Autodesk Fusion 360 part; units mm, degrees
(part 2 of 3)
  measures "d264" distance of L157.end L157.start
  measures "d265" distance of L181.start L179.start
  measures "d266" distance of L180.end L182.end
  measures "d267" distance of L180.start L179.end
  measures "d268" distance of L154.end L154.start
  measures "d269" distance of L174.end L171.start
  measures "d270" distance of L153.start L154.end
  measures "d271" distance of L162.end L156.end
  measures "d272" distance of L156.start L156.end
  measures "d273" distance of L156 L187
  measures "d274" distance of L159.start L161.end
  measures "d275" distance of L158 L163
  measures "d276" distance of L158.end L153.end
  measures "d277" distance of L162.end L168.end
  measures "d278" distance of L157.end L165.end
  measures "d279" distance of L167.start L167.end
  measures "d280" distance of L190.end L189.end
  measures "d281" distance of L190.end L191.end
  measures "d282" distance of L194.start L195.end
  measures "d283" distance of L193.start L194.start
  measures "d284" distance of L192 L196
  measures "d285" distance of L187 L194
  measures "d286" distance of P0 L196
  measures "d287" distance of L200.start L197.end
  measures "d288" distance of L200.end L200.start
  measures "d289" distance of L198.start L198.end
  measures "d290" distance of L198.end L199.start
  measures "d291" distance of L198 L203
  measures "d292" distance of L205.end L207.end
  measures "d293" distance of L206.start L207.end
  measures "d294" distance of L202 L206
  measures "d295" distance of L212.end L214.end
  measures "d296" distance of L216.start L214.end
  measures "d297" distance of L217.start L215.end
  measures "d298" distance of L217.end L217.start
  measures "d300" distance of L210.end L209.start
  measures "d301" distance of L209.end L209.start
  measures "d303" distance of L200 L212
  measures "d305" distance of L156 L197
  measures "d306" distance of L221.end L221.start
  measures "d307" distance of L221.end L223.start
  measures "d312" distance of L242.end L237.end
  measures "d313" distance of L236.end L237.end
  measures "d314" distance of L236.end L236.start
  measures "d315" distance of L238.start L255.start
  measures "d316" distance of L241.end L244.start
  measures "d317" distance of L243.end L250.end
  measures "d318" distance of L239.end L239.start
  measures "d319" distance of L230.end L225.start
  measures "d320" distance of L229.start L232.start
  measures "d321" distance of L225.end L225.start
  measures "d322" distance of L249.start L231.end
  measures "d323" distance of L231.end L231.start
  measures "d324" distance of L231 L245
  measures "d325" distance of L234.end L236.start
  measures "d326" distance of L248 L256
  measures "d327" distance of L226.end L234.start
  measures "d328" distance of L249.start L230.start
  measures "d329" distance of L238.start L238.end
  measures "d330" distance of L251.end L245.start
  measures "d375" distance of L272.start L267.end
  measures "d376" distance of L264.end L267.end
  measures "d377" distance of L264.end L264.start
  measures "d378" distance of L261.start L266.start
  measures "d379" distance of L274.start L274.end
  measures "d380" distance of L276.start L276.end
  measures "d381" distance of L283.end L277.end
  measures "d382" distance of L269.end L269.start
  measures "d383" distance of L284.start L284.end
  measures "d384" distance of L270.end L269.end
  measures "d385" distance of L262.end L262.start
  measures "d386" distance of L275.end L262.start
  measures "d387" distance of L289 L290
  measures "d388" distance of L264.start L265.start
  measures "d389" distance of L265 L268
  measures "d390" distance of L268.end L268.start
  measures "d391" distance of L262.end L271.end
  measures "d392" distance of L261.start L261.end
  measures "d393" distance of L263.end L289.start
  measures "d395" distance of origin L220
  measures "d399" angle of L30 L221
  measures "d401" distance of L221 L297
  measures "d402" distance of L30 P2
  measures "d403" distance of L29 P2
  measures "d404" distance of L297 P2
  measures "d405" distance of L223 L298
  measures "d407" angle of L223 L233
  measures "d408" distance of L231 P5
  measures "d409" distance of L240 P5
  measures "d410" distance of L298 P5
  measures "d411" distance of L231 P6
  measures "d412" distance of L260 P6
  measures "d413" distance of L289 L304
  measures "d414" distance of P6 L304
  measures "d415" distance of L127 L305
  measures "d416" distance of L132 L306
  measures "d418" angle of L248 L289
  measures "d419" distance of L289 L307
  measures "d420" distance of L293 L308
  measures "d421" distance of L306 L307.end
  measures "d423" distance of L8 L309
  measures "d424" distance of L63 L310
  measures "d494" angle of L87 L314
  measures "d496" distance of L213 L314
  measures "d497" distance of L77 P7
  measures "d498" distance of L218 L315
  measures "d499" distance of L195 L317
  measures "d512" distance of L224 L319
  measures "d543" diameter of A3
  measures "d544" diameter of A4
  measures "d545" diameter of A5
  measures "d546" diameter of A6
  measures "d547" diameter of A7
  measures "d548" diameter of A8
  measures "d550" diameter of A9
  measures "d551" diameter of A10
  measures "d553" diameter of A11
  measures "d554" diameter of A12
  measures "d555" diameter of A13
  measures "d556" diameter of A14
  measures "d557" distance of L314 A11.centre
  measures "d558" distance of L315 A13.centre
  measures "d587" diameter of A15
  measures "d588" diameter of A16
  measures "d589" diameter of A17
  measures "d590" diameter of A18
  measures "d591" diameter of A19
  measures "d592" diameter of A20
  measures "d593" diameter of A21
  measures "d594" diameter of A22
  measures "d595" diameter of A23
  measures "d596" diameter of A24
  measures "d597" diameter of A25
  measures "d598" diameter of A26
  measures "d599" diameter of A27
  measures "d600" diameter of A28
  measures "d601" diameter of A29
  measures "d602" diameter of A30
  measures "d603" diameter of A31
  measures "d604" diameter of A32
  measures "d605" diameter of A33
  measures "d606" diameter of A34
  measures "d607" diameter of A35
  measures "d608" diameter of A36
  measures "d609" diameter of A37
  measures "d610" diameter of A38
  measures "d611" angle of L309 L317
  measures "d617" angle of L190 L334
  measures "d618" angle of L193 L335
  measures "d620" vertical distance of A5.centre A7.centre
  measures "d621" distance of A5.centre L322
  measures "d645" diameter of A39
  measures "d649" diameter of A40
  measures "d651" diameter of A41
  measures "d653" diameter of A42
  measures "d655" diameter of A43
  measures "d657" diameter of A44
  measures "d661" diameter of A45
  measures "d662" diameter of A46
  measures "d663" diameter of A47
  measures "d664" diameter of A48
  measures "d665" diameter of A49
  measures "d666" diameter of A50
  measures "d667" diameter of A51
  measures "d668" diameter of A52
  measures "d669" diameter of A53
  measures "d670" diameter of A54
  measures "d671" diameter of A55
  measures "d672" diameter of A56
  measures "d705" diameter of A62
  measures "d706" diameter of A61
  measures "d707" diameter of A58
  measures "d708" diameter of A57
  measures "d709" diameter of A60
  measures "d710" diameter of A59
extrude "Platte Rechts" add sketch "Skizze1" along normal blind 2.7 contours L309 L310 L311 A0 L314 A1 A2 L318 | A15 | A16 | A17 | A18 | A19 | A20 | A21 | A22 | A23 | A24 | A25 | A26 | A27 | A28 | A29 | A30 | A31 | A32 | A33 | A34 | A35 | A36 | A37 | A38 | A45 | A46 | A47 | A48 | A49 | A50 | A51 | A52 | A53 | A54 | A55 | A56 makes body 1
extrude "Platte Mitte" add sketch "Skizze1" along normal blind 2.7 separate body contours L313 L314 L315 L316 L317 | A3 | A4 | A5 | A6 | A7 | A8 | A9 | A10 | A11 | A12 | A13 | A14 | A39 | A40 | A41 | A42 | A43 | A44 | A57 | A58 | A59 | A60 | A61 | A62 makes body 2
sketch "Skizze5" plane through (0, 0, 0) normal (1, 0, 0) x (0, 1, 0)
  line L0 (0, 12.7887) -> (160, 19.7745)
  line L1 (0, 1.75) -> (0, 22.5)
  line L2 (1.75, 0) -> (22.5, 0)
  point P0 (14, 13.4)
  dimension "d440" = 2.5
  dimension "d441" = 160
  dimension "d450" = 14
  dimension "d451" = 13.4
  constraint coincident L0.start L1
  constraint coincident L0 P0
  measures "d440" angle of L0 L2
  measures "d441" distance of L0.end L1
  measures "d450" distance of L1 P0
  measures "d451" distance of L2 P0
ref_plane "Arbeitsebene1" through (0, 80, 16.2816) normal (0, 0.043619, -0.999048) x (0, 0.999048, 0.043619)
sketch "Skizze4" plane through (0, 0, 2.7) normal (0, 0, 1) x (-1, 0, 0)
  line L0 (97.7927, -100.387) -> (100.2238, -86.5997)
  line L1 (100.2238, -86.5997) -> (114.0111, -89.0308)
  line L2 (114.0111, -89.0308) -> (111.58, -102.8181)
  line L3 (111.58, -102.8181) -> (97.7927, -100.387)
  line L4 (133.2058, -89.8768) -> (130.7747, -103.6641)
  line L5 (130.7747, -103.6641) -> (116.9874, -101.233)
  line L6 (116.9874, -101.233) -> (119.4185, -87.4457)
  line L7 (119.4185, -87.4457) -> (133.2058, -89.8768)
  line L8 (96.9158, -105.3603) -> (110.7031, -107.7914)
  line L9 (110.7031, -107.7914) -> (108.272, -121.5787)
  line L10 (108.272, -121.5787) -> (94.4847, -119.1476)
  line L11 (94.4847, -119.1476) -> (96.9158, -105.3603)
  line L12 (110.3714, -138.7542) -> (112.8025, -124.9669)
  line L13 (112.8025, -124.9669) -> (126.5898, -127.3979)
  line L14 (126.5898, -127.3979) -> (124.1587, -141.1852)
  line L15 (124.1587, -141.1852) -> (110.3714, -138.7542)
  line L16 (107.3951, -126.552) -> (104.964, -140.3393)
  line L17 (104.964, -140.3393) -> (91.1767, -137.9082)
  line L18 (91.1767, -137.9082) -> (93.6078, -124.1209)
  line L19 (93.6078, -124.1209) -> (107.3951, -126.552)
  line L20 (156.9327, -65.0193) -> (143.1454, -62.5882)
  line L21 (143.1454, -62.5882) -> (145.5765, -48.8009)
  line L22 (145.5765, -48.8009) -> (159.3638, -51.232)
  line L23 (159.3638, -51.232) -> (156.9327, -65.0193)
  line L24 (39.3317, -102.8224) -> (41.7627, -89.0351)
  line L25 (41.7627, -89.0351) -> (55.55, -91.4661)
  line L26 (55.55, -91.4661) -> (53.119, -105.2534)
  line L27 (53.119, -105.2534) -> (39.3317, -102.8224)
  line L28 (78.5893, -99.5903) -> (92.3766, -102.0214)
  line L29 (92.3766, -102.0214) -> (89.9455, -115.8087)
  line L30 (89.9455, -115.8087) -> (76.1582, -113.3776)
  line L31 (76.1582, -113.3776) -> (78.5893, -99.5903)
  line L32 (56.868, -113.0733) -> (70.6553, -115.5043)
  line L33 (70.6553, -115.5043) -> (68.2243, -129.2916)
  line L34 (68.2243, -129.2916) -> (54.437, -126.8606)
  line L35 (54.437, -126.8606) -> (56.868, -113.0733)
  line L36 (52.242, -110.2267) -> (49.811, -124.014)
  line L37 (49.811, -124.014) -> (36.0237, -121.583)
  line L38 (36.0237, -121.583) -> (38.4547, -107.7956)
  line L39 (38.4547, -107.7956) -> (52.242, -110.2267)
  line L40 (75.2813, -118.3509) -> (89.0686, -120.7819)
  line L41 (89.0686, -120.7819) -> (86.6376, -134.5693)
  line L42 (86.6376, -134.5693) -> (72.8502, -132.1382)
  line L43 (72.8502, -132.1382) -> (75.2813, -118.3509)
  line L44 (57.7449, -108.1) -> (60.176, -94.3127)
  line L45 (60.176, -94.3127) -> (73.9633, -96.7437)
  line L46 (73.9633, -96.7437) -> (71.5323, -110.5311)
  line L47 (71.5323, -110.5311) -> (57.7449, -108.1)
  line L48 (81.8973, -80.8297) -> (95.6846, -83.2608)
  line L49 (95.6846, -83.2608) -> (93.2535, -97.0481)
  line L50 (93.2535, -97.0481) -> (79.4662, -94.617)
  line L51 (79.4662, -94.617) -> (81.8973, -80.8297)
  line L52 (63.484, -75.5521) -> (77.2713, -77.9832)
  line L53 (77.2713, -77.9832) -> (74.8403, -91.7705)
  line L54 (74.8403, -91.7705) -> (61.0529, -89.3394)
  line L55 (61.0529, -89.3394) -> (63.484, -75.5521)
  line L56 (66.792, -56.7915) -> (80.5793, -59.2226)
  line L57 (80.5793, -59.2226) -> (78.1483, -73.0099)
  line L58 (78.1483, -73.0099) -> (64.3609, -70.5788)
  line L59 (64.3609, -70.5788) -> (66.792, -56.7915)
  line L60 (85.2053, -62.0691) -> (98.9926, -64.5002)
  line L61 (98.9926, -64.5002) -> (96.5615, -78.2875)
  line L62 (96.5615, -78.2875) -> (82.7742, -75.8564)
  line L63 (82.7742, -75.8564) -> (85.2053, -62.0691)
  line L64 (56.4175, -85.2219) -> (50.228, -84.1305)
  line L65 (50.228, -84.1305) -> (50.0847, -84.943)
  line L66 (50.0847, -84.943) -> (47.3421, -84.4594)
  line L67 (47.3421, -84.4594) -> (47.4853, -83.6469)
  line L68 (47.4853, -83.6469) -> (44.3044, -83.086)
  line L69 (44.3044, -83.086) -> (45.4765, -76.4386)
  line L70 (45.4765, -76.4386) -> (48.6574, -76.9995)
  line L71 (48.6574, -76.9995) -> (48.9223, -75.4976)
  line L72 (48.9223, -75.4976) -> (44.2937, -74.6815)
  line L73 (44.2937, -74.6815) -> (46.7247, -60.8942)
  line L74 (46.7247, -60.8942) -> (51.3533, -61.7103)
  line L75 (51.3533, -61.7103) -> (51.6181, -60.2085)
  line L76 (51.6181, -60.2085) -> (48.4372, -59.6476)
  line L77 (48.4372, -59.6476) -> (49.6093, -53.0002)
  line L78 (49.6093, -53.0002) -> (52.7903, -53.561)
  line L79 (52.7903, -53.561) -> (52.9335, -52.7486)
  line L80 (52.9335, -52.7486) -> (55.6762, -53.2322)
  line L81 (55.6762, -53.2322) -> (55.533, -54.0446)
  line L82 (55.533, -54.0446) -> (61.7225, -55.136)
  line L83 (61.7225, -55.136) -> (61.4229, -56.8348)
  line L84 (61.4229, -56.8348) -> (62.6047, -57.0432)
  line L85 (62.6047, -57.0432) -> (62.0317, -60.2931)
  line L86 (62.0317, -60.2931) -> (60.8499, -60.0847)
  line L87 (60.8499, -60.0847) -> (60.5503, -61.7835)
  line L88 (60.5503, -61.7835) -> (56.1483, -61.0073)
  line L89 (56.1483, -61.0073) -> (55.8834, -62.5091)
  line L90 (55.8834, -62.5091) -> (60.512, -63.3252)
  line L91 (60.512, -63.3252) -> (58.081, -77.1126)
  line L92 (58.081, -77.1126) -> (53.4524, -76.2964)
  line L93 (53.4524, -76.2964) -> (53.1876, -77.7982)
  line L94 (53.1876, -77.7982) -> (57.5896, -78.5744)
  line L95 (57.5896, -78.5744) -> (57.2901, -80.2732)
  line L96 (57.2901, -80.2732) -> (58.4719, -80.4816)
  line L97 (58.4719, -80.4816) -> (57.8988, -83.7315)
  line L98 (57.8988, -83.7315) -> (56.7171, -83.5231)
  line L99 (56.7171, -83.5231) -> (56.4175, -85.2219)
  line L100 (109.906, -37.6121) -> (123.0617, -42.4003)
  line L101 (123.0617, -42.4003) -> (118.2734, -55.556)
  line L102 (118.2734, -55.556) -> (105.1177, -50.7677)
  line L103 (105.1177, -50.7677) -> (109.906, -37.6121)
  line L104 (79.2965, -35.8234) -> (81.6465, -31.753)
  line L105 (81.6465, -31.753) -> (93.7709, -38.753)
  line L106 (93.7709, -38.753) -> (91.4209, -42.8234)
  line L107 (91.4209, -42.8234) -> (92.7416, -43.5859)
  line L108 (92.7416, -43.5859) -> (94.3566, -40.7886)
  line L109 (94.3566, -40.7886) -> (100.2022, -44.1636)
  line L110 (100.2022, -44.1636) -> (98.5872, -46.9609)
  line L111 (98.5872, -46.9609) -> (99.3017, -47.3734)
  line L112 (99.3017, -47.3734) -> (97.9092, -49.7852)
  line L113 (97.9092, -49.7852) -> (97.1947, -49.3727)
  line L114 (97.1947, -49.3727) -> (94.0522, -54.8157)
  line L115 (94.0522, -54.8157) -> (92.5583, -53.9532)
  line L116 (92.5583, -53.9532) -> (91.9583, -54.9924)
  line L117 (91.9583, -54.9924) -> (89.1005, -53.3424)
  line L118 (89.1005, -53.3424) -> (89.7005, -52.3032)
  line L119 (89.7005, -52.3032) -> (88.2066, -51.4407)
  line L120 (88.2066, -51.4407) -> (90.4416, -47.5696)
  line L121 (90.4416, -47.5696) -> (89.1209, -46.8071)
  line L122 (89.1209, -46.8071) -> (86.7709, -50.8774)
  line L123 (86.7709, -50.8774) -> (74.6465, -43.8774)
  line L124 (74.6465, -43.8774) -> (76.9965, -39.8071)
  line L125 (76.9965, -39.8071) -> (75.6758, -39.0446)
  line L126 (75.6758, -39.0446) -> (73.4408, -42.9157)
  line L127 (73.4408, -42.9157) -> (71.9469, -42.0532)
  line L128 (71.9469, -42.0532) -> (71.3469, -43.0924)
  line L129 (71.3469, -43.0924) -> (68.4891, -41.4424)
  line L130 (68.4891, -41.4424) -> (69.0891, -40.4032)
  line L131 (69.0891, -40.4032) -> (67.5952, -39.5407)
  line L132 (67.5952, -39.5407) -> (70.7377, -34.0977)
  line L133 (70.7377, -34.0977) -> (70.0232, -33.6852)
  line L134 (70.0232, -33.6852) -> (71.4157, -31.2734)
  line L135 (71.4157, -31.2734) -> (72.1302, -31.6859)
  line L136 (72.1302, -31.6859) -> (73.7452, -28.8886)
  line L137 (73.7452, -28.8886) -> (79.5908, -32.2636)
  line L138 (79.5908, -32.2636) -> (77.9758, -35.0609)
  line L139 (77.9758, -35.0609) -> (79.2965, -35.8234)
  line L140 (43.5918, -39.6557) -> (44.1221, -39.0237)
  line L141 (44.1221, -39.0237) -> (41.6478, -36.9475)
  line L142 (41.6478, -36.9475) -> (45.9866, -31.7767)
  line L143 (45.9866, -31.7767) -> (48.461, -33.8529)
  line L144 (48.461, -33.8529) -> (49.4412, -32.6847)
  line L145 (49.4412, -32.6847) -> (45.8408, -29.6636)
  line L146 (45.8408, -29.6636) -> (54.8398, -18.939)
  line L147 (54.8398, -18.939) -> (58.4402, -21.9601)
  line L148 (58.4402, -21.9601) -> (59.4205, -20.7919)
  line L149 (59.4205, -20.7919) -> (56.9462, -18.7157)
  line L150 (56.9462, -18.7157) -> (61.285, -13.5449)
  line L151 (61.285, -13.5449) -> (63.7593, -15.6211)
  line L152 (63.7593, -15.6211) -> (64.2896, -14.9891)
  line L153 (64.2896, -14.9891) -> (66.423, -16.7793)
  line L154 (66.423, -16.7793) -> (65.8927, -17.4113)
  line L155 (65.8927, -17.4113) -> (70.7073, -21.4512)
  line L156 (70.7073, -21.4512) -> (69.5985, -22.7726)
  line L157 (69.5985, -22.7726) -> (70.5178, -23.5439)
  line L158 (70.5178, -23.5439) -> (68.3966, -26.0719)
  line L159 (68.3966, -26.0719) -> (67.4773, -25.3005)
  line L160 (67.4773, -25.3005) -> (66.3685, -26.622)
  line L161 (66.3685, -26.622) -> (62.9443, -23.7487)
  line L162 (62.9443, -23.7487) -> (61.964, -24.9169)
  line L163 (61.964, -24.9169) -> (65.5644, -27.938)
  line L164 (65.5644, -27.938) -> (56.5654, -38.6627)
  line L165 (56.5654, -38.6627) -> (52.965, -35.6416)
  line L166 (52.965, -35.6416) -> (51.9848, -36.8098)
  line L167 (51.9848, -36.8098) -> (55.409, -39.683)
  line L168 (55.409, -39.683) -> (54.3002, -41.0045)
  line L169 (54.3002, -41.0045) -> (55.2194, -41.7758)
  line L170 (55.2194, -41.7758) -> (53.0982, -44.3037)
  line L171 (53.0982, -44.3037) -> (52.179, -43.5324)
  line L172 (52.179, -43.5324) -> (51.0702, -44.8538)
  line L173 (51.0702, -44.8538) -> (46.2556, -40.8139)
  line L174 (46.2556, -40.8139) -> (45.7253, -41.4459)
  line L175 (45.7253, -41.4459) -> (43.5918, -39.6557)
  line L176 (153.6247, -83.7798) -> (139.8374, -81.3488)
  line L177 (139.8374, -81.3488) -> (142.2685, -67.5615)
  line L178 (142.2685, -67.5615) -> (156.0558, -69.9925)
  line L179 (156.0558, -69.9925) -> (153.6247, -83.7798)
  line L180 (129.8978, -108.6374) -> (127.4667, -122.4247)
  line L181 (127.4667, -122.4247) -> (113.6794, -119.9936)
  line L182 (113.6794, -119.9936) -> (116.1105, -106.2063)
  line L183 (116.1105, -106.2063) -> (129.8978, -108.6374)
  line L184 (136.5138, -71.1162) -> (134.0827, -84.9035)
  line L185 (134.0827, -84.9035) -> (120.2954, -82.4724)
  line L186 (120.2954, -82.4724) -> (122.7265, -68.6851)
  line L187 (122.7265, -68.6851) -> (136.5138, -71.1162)
  line L188 (171.5084, -92.0611) -> (169.0773, -105.8484)
  line L189 (169.0773, -105.8484) -> (155.29, -103.4174)
  line L190 (155.29, -103.4174) -> (157.7211, -89.6301)
  line L191 (157.7211, -89.6301) -> (171.5084, -92.0611)
  line L192 (129.9134, -137.6305) -> (132.3445, -123.8432)
  line L193 (132.3445, -123.8432) -> (146.1318, -126.2743)
  line L194 (146.1318, -126.2743) -> (143.7007, -140.0616)
  line L195 (143.7007, -140.0616) -> (129.9134, -137.6305)
  line L196 (158.598, -84.6568) -> (161.0291, -70.8695)
  line L197 (161.0291, -70.8695) -> (174.8164, -73.3005)
  line L198 (174.8164, -73.3005) -> (172.3853, -87.0878)
  line L199 (172.3853, -87.0878) -> (158.598, -84.6568)
  line L200 (164.8924, -129.5823) -> (162.4613, -143.3696)
  line L201 (162.4613, -143.3696) -> (148.674, -140.9385)
  line L202 (148.674, -140.9385) -> (151.1051, -127.1512)
  line L203 (151.1051, -127.1512) -> (164.8924, -129.5823)
  line L204 (149.4398, -107.5137) -> (147.0087, -121.301)
  line L205 (147.0087, -121.301) -> (133.2214, -118.8699)
  line L206 (133.2214, -118.8699) -> (135.6525, -105.0826)
  line L207 (135.6525, -105.0826) -> (149.4398, -107.5137)
  line L208 (168.2004, -110.8217) -> (165.7693, -124.609)
  line L209 (165.7693, -124.609) -> (151.982, -122.1779)
  line L210 (151.982, -122.1779) -> (154.4131, -108.3906)
  line L211 (154.4131, -108.3906) -> (168.2004, -110.8217)
  line L212 (138.9605, -86.3221) -> (152.7478, -88.7531)
  line L213 (152.7478, -88.7531) -> (150.3167, -102.5404)
  line L214 (150.3167, -102.5404) -> (136.5294, -100.1094)
  line L215 (136.5294, -100.1094) -> (138.9605, -86.3221)
  line L216 (175.6933, -68.3273) -> (161.906, -65.8962)
  line L217 (161.906, -65.8962) -> (164.3371, -52.1089)
  line L218 (164.3371, -52.1089) -> (178.1244, -54.5399)
  line L219 (178.1244, -54.5399) -> (175.6933, -68.3273)
  line L220 (117.3191, -70.2702) -> (114.888, -84.0575)
  line L221 (114.888, -84.0575) -> (101.1007, -81.6264)
  line L222 (101.1007, -81.6264) -> (103.5318, -67.8391)
  line L223 (103.5318, -67.8391) -> (117.3191, -70.2702)
  line L224 (139.8218, -52.3556) -> (137.3907, -66.1429)
  line L225 (137.3907, -66.1429) -> (123.6034, -63.7118)
  line L226 (123.6034, -63.7118) -> (126.0345, -49.9245)
  line L227 (126.0345, -49.9245) -> (139.8218, -52.3556)
  line L228 (166.5386, -157.8222) -> (185.963, -47.6611)
  line L229 (185.963, -47.6611) -> (142.0159, -39.9121)
  arc A0 (71.1177, -6.8517) -> (142.0159, -39.9121) centre (168.2583, 108.916) ccw
  line L230 (33.7619, -134.4101) -> (166.5386, -157.8222)
  line L231 (164.3485, -154.6944) -> (34.2307, -131.7511)
  line L232 (164.3485, -154.6944) -> (182.8351, -49.8513)
  line L233 (182.8351, -49.8513) -> (141.5471, -42.5711)
  line L234 (33.7619, -134.4101) -> (34.2307, -131.7511) construction
  line L235 (142.0159, -39.9121) -> (141.5471, -42.5711) construction
  line L236 (0, -2.5) -> (0, -20)
  arc A1 (71.1177, -6.8517) -> (52.2928, 0) centre (52.2928, -29.2863) ccw
  line L237 (52.2928, 0) -> (31.075, 0)
  line L238 (31.075, 0) -> (31.075, -134.175)
  arc A2 (33.7619, -134.4101) -> (31.075, -134.175) centre (31.075, -149.6482) ccw
  line L239 (52.2928, -2.7) -> (32.425, -2.7)
  line L240 (32.425, -2.7) -> (32.425, -131.4327)
  line L241 (52.2928, -2.7) -> (52.2928, 0) construction
  line L242 (34.2307, -131.7511) -> (32.425, -131.4327)
  line L243 (29.725, -131.475) -> (-29.725, -131.475)
  line L244 (-29.725, -131.475) -> (-29.725, -2.7)
  line L245 (-29.725, -2.7) -> (29.725, -2.7)
  line L246 (29.725, -2.7) -> (29.725, -131.475)
  line L247 (-31.075, 0) -> (-31.075, -134.175)
  line L248 (-31.075, -134.175) -> (31.075, -134.175)
  line L249 (26.05, -50) -> (26.05, -64)
  arc A3 (69.3822, -8.92) -> (141.5471, -42.5711) centre (168.2583, 108.916) ccw
  arc A4 (69.3822, -8.92) -> (52.2928, -2.7) centre (52.2928, -29.2863) ccw
  line L250 (71.1177, -6.8517) -> (69.3822, -8.92) construction
  line L251 (31.075, 0) -> (-31.075, 0)
  line L252 (-12.025, -121.15) -> (-12.025, -122.15)
  line L253 (-12.025, -122.15) -> (-7.025, -122.15)
  line L254 (-7.025, -122.15) -> (-7.025, -121.15)
  line L255 (-2.525, -121.15) -> (-16.525, -121.15) construction
  line L256 (-2.525, -107.15) -> (-2.525, -121.15) construction
  line L257 (-12.025, -121.15) -> (-7.025, -121.15)
  line L258 (-12.025, -107.15) -> (-7.025, -107.15)
  line L259 (-7.025, -107.15) -> (-7.025, -106.15)
  line L260 (-7.025, -106.15) -> (-12.025, -106.15)
  line L261 (-12.025, -106.15) -> (-12.025, -107.15)
  line L262 (7.025, -121.15) -> (12.025, -121.15)
  line L263 (12.025, -121.15) -> (12.025, -122.15)
  line L264 (12.025, -122.15) -> (7.025, -122.15)
  line L265 (7.025, -122.15) -> (7.025, -121.15)
  line L266 (7.025, -107.15) -> (12.025, -107.15)
  line L267 (12.025, -107.15) -> (12.025, -106.15)
  line L268 (12.025, -106.15) -> (7.025, -106.15)
  line L269 (7.025, -106.15) -> (7.025, -107.15)
  line L270 (-21.55, -83.05) -> (-16.55, -83.05)
  line L271 (-16.55, -83.05) -> (-16.55, -84.05)
  line L272 (-16.55, -84.05) -> (-21.55, -84.05)
  line L273 (-21.55, -84.05) -> (-21.55, -83.05)
  line L274 (-12.05, -83.05) -> (-26.05, -83.05)
  line L275 (-12.05, -69.05) -> (-12.05, -83.05)
  line L276 (-21.55, -69.05) -> (-16.55, -69.05)
  line L277 (-16.55, -69.05) -> (-16.55, -68.05)
  line L278 (-16.55, -68.05) -> (-21.55, -68.05)
  line L279 (-21.55, -68.05) -> (-21.55, -69.05)
  line L280 (-2.5, -83.05) -> (2.5, -83.05)
  line L281 (2.5, -83.05) -> (2.5, -84.05)
  line L282 (2.5, -84.05) -> (-2.5, -84.05)
  line L283 (-2.5, -84.05) -> (-2.5, -83.05)
  line L284 (-2.5, -69.05) -> (2.5, -69.05)
  line L285 (2.5, -69.05) -> (2.5, -68.05)
  line L286 (2.5, -68.05) -> (-2.5, -68.05)
  line L287 (-2.5, -68.05) -> (-2.5, -69.05)
  line L288 (16.55, -83.05) -> (21.55, -83.05)
  line L289 (21.55, -83.05) -> (21.55, -84.05)
  line L290 (21.55, -84.05) -> (16.55, -84.05)
  line L291 (16.55, -84.05) -> (16.55, -83.05)
  line L292 (16.55, -69.05) -> (21.55, -69.05)
  line L293 (21.55, -69.05) -> (21.55, -68.05)
  line L294 (21.55, -68.05) -> (16.55, -68.05)
  line L295 (16.55, -68.05) -> (16.55, -69.05)
  line L296 (-21.55, -64) -> (-16.55, -64)
  line L297 (-16.55, -64) -> (-16.55, -65)
  line L298 (-16.55, -65) -> (-21.55, -65)
  line L299 (-21.55, -65) -> (-21.55, -64)
  line L300 (-12.05, -64) -> (-26.05, -64)
  line L301 (-2.5, -64) -> (2.5, -64)
  line L302 (2.5, -64) -> (2.5, -65)
  line L303 (2.5, -65) -> (-2.5, -65)
  line L304 (-2.5, -65) -> (-2.5, -64)
  line L305 (16.55, -64) -> (21.55, -64)
  line L306 (21.55, -64) -> (21.55, -65)
  line L307 (21.55, -65) -> (16.55, -65)
  line L308 (16.55, -65) -> (16.55, -64)
  line L309 (-21.55, -50) -> (-16.55, -50)
  line L310 (-16.55, -50) -> (-16.55, -49)
  line L311 (-16.55, -49) -> (-21.55, -49)
  line L312 (-21.55, -49) -> (-21.55, -50)
  line L313 (-2.5, -50) -> (2.5, -50)
  line L314 (2.5, -50) -> (2.5, -49)
  line L315 (2.5, -49) -> (-2.5, -49)
  line L316 (-2.5, -49) -> (-2.5, -50)
  line L317 (16.55, -50) -> (21.55, -50)
  line L318 (21.55, -50) -> (21.55, -49)
  line L319 (21.55, -49) -> (16.55, -49)
  line L320 (16.55, -49) -> (16.55, -50)
  line L321 (46.368, -88.8317) -> (51.2921, -89.6999)
  line L322 (51.2921, -89.6999) -> (51.1184, -90.6847)
  line L323 (51.1184, -90.6847) -> (46.1944, -89.8165)
  line L324 (46.1944, -89.8165) -> (46.368, -88.8317)
  line L325 (48.6873, -104.472) -> (48.5137, -105.4568)
  line L326 (43.7633, -103.6038) -> (48.6873, -104.472)
  line L327 (43.5896, -104.5886) -> (43.7633, -103.6038)
  line L328 (48.5137, -105.4568) -> (43.5896, -104.5886)
  line L329 (47.9841, -108.4605) -> (47.8104, -109.4453)
  line L330 (43.06, -107.5923) -> (47.9841, -108.4605)
  line L331 (42.8864, -108.5771) -> (43.06, -107.5923)
  line L332 (47.8104, -109.4453) -> (42.8864, -108.5771)
  line L333 (45.3793, -123.2326) -> (45.2057, -124.2174)
  line L334 (40.4553, -122.3644) -> (45.3793, -123.2326)
  line L335 (40.2816, -123.3492) -> (40.4553, -122.3644)
  line L336 (45.2057, -124.2174) -> (40.2816, -123.3492)
  line L337 (58.6949, -128.6268) -> (58.8686, -127.642)
  line L338 (63.619, -129.495) -> (58.6949, -128.6268)
  line L339 (63.7926, -128.5102) -> (63.619, -129.495)
  line L340 (58.8686, -127.642) -> (63.7926, -128.5102)
  line L341 (61.2997, -113.8547) -> (61.4733, -112.8699)
  line L342 (61.4733, -112.8699) -> (66.3973, -113.7381)
  line L343 (66.2237, -114.7229) -> (61.2997, -113.8547)
  line L344 (66.3973, -113.7381) -> (66.2237, -114.7229)
  line L345 (67.1006, -109.7496) -> (66.927, -110.7344)
  line L346 (66.927, -110.7344) -> (62.0029, -109.8662)
  line L347 (62.1766, -108.8814) -> (67.1006, -109.7496)
  line L348 (62.0029, -109.8662) -> (62.1766, -108.8814)
  line L349 (64.6077, -95.0941) -> (64.7813, -94.1093)
  line L350 (64.7813, -94.1093) -> (69.7053, -94.9775)
  line L351 (69.7053, -94.9775) -> (69.5317, -95.9623)
  line L352 (69.5317, -95.9623) -> (64.6077, -95.0941)
  line L353 (65.3109, -91.1056) -> (65.4846, -90.1208)
  line L354 (70.235, -91.9739) -> (65.3109, -91.1056)
  line L355 (70.4086, -90.989) -> (70.235, -91.9739)
  line L356 (65.4846, -90.1208) -> (70.4086, -90.989)
  line L357 (67.9157, -76.3335) -> (68.0893, -75.3487)
  line L358 (68.0893, -75.3487) -> (73.0133, -76.2169)
  line L359 (72.8397, -77.2017) -> (67.9157, -76.3335)
  line L360 (73.0133, -76.2169) -> (72.8397, -77.2017)
  line L361 (73.7166, -72.2285) -> (73.543, -73.2133)
  line L362 (73.543, -73.2133) -> (68.6189, -72.345)
  line L363 (68.7926, -71.3602) -> (73.7166, -72.2285)
  line L364 (68.6189, -72.345) -> (68.7926, -71.3602)
  line L365 (71.2237, -57.5729) -> (71.3973, -56.5881)
  line L366 (71.3973, -56.5881) -> (76.3213, -57.4563)
  line L367 (76.3213, -57.4563) -> (76.1477, -58.4412)
  line L368 (76.1477, -58.4412) -> (71.2237, -57.5729)
  line L369 (77.2819, -132.9196) -> (82.2059, -133.7878)
  line L370 (77.1082, -133.9044) -> (77.2819, -132.9196)
  line L371 (82.2059, -133.7878) -> (82.0323, -134.7726)
  line L372 (82.0323, -134.7726) -> (77.1082, -133.9044)
  line L373 (79.713, -119.1323) -> (79.8866, -118.1475)
  line L374 (84.637, -120.0005) -> (79.713, -119.1323)
  line L375 (84.8106, -119.0157) -> (84.637, -120.0005)
  line L376 (79.8866, -118.1475) -> (84.8106, -119.0157)
  line L377 (85.3403, -116.0121) -> (80.4162, -115.1438)
  line L378 (85.5139, -115.0272) -> (85.3403, -116.0121)
  line L379 (80.5899, -114.159) -> (85.5139, -115.0272)
  line L380 (80.4162, -115.1438) -> (80.5899, -114.159)
  line L381 (88.1186, -100.2551) -> (87.945, -101.2399)
  line L382 (83.1946, -99.3869) -> (88.1186, -100.2551)
  line L383 (87.945, -101.2399) -> (83.0209, -100.3717)
  line L384 (83.0209, -100.3717) -> (83.1946, -99.3869)
  line L385 (83.7242, -96.3832) -> (83.8979, -95.3984)
  line L386 (88.6483, -97.2515) -> (83.7242, -96.3832)
  line L387 (88.8219, -96.2667) -> (88.6483, -97.2515)
  line L388 (83.8979, -95.3984) -> (88.8219, -96.2667)
  line L389 (86.5026, -80.6263) -> (91.4266, -81.4945)
  line L390 (91.253, -82.4794) -> (86.3289, -81.6111)
  line L391 (91.4266, -81.4945) -> (91.253, -82.4794)
  line L392 (86.3289, -81.6111) -> (86.5026, -80.6263)
  line L393 (87.0322, -77.6226) -> (87.2059, -76.6378)
  line L394 (91.9563, -78.4909) -> (87.0322, -77.6226)
  line L395 (92.1299, -77.5061) -> (91.9563, -78.4909)
  line L396 (87.2059, -76.6378) -> (92.1299, -77.5061)
  line L397 (89.6369, -62.8505) -> (89.8106, -61.8657)
  line L398 (94.561, -63.7188) -> (89.6369, -62.8505)
  line L399 (94.7346, -62.734) -> (94.561, -63.7188)
  line L400 (89.8106, -61.8657) -> (94.7346, -62.734)
  line L401 (95.6083, -138.6896) -> (100.5324, -139.5579)
  line L402 (95.4347, -139.6744) -> (95.6083, -138.6896)
  line L403 (100.5324, -139.5579) -> (100.3587, -140.5427)
  line L404 (100.3587, -140.5427) -> (95.4347, -139.6744)
  line L405 (98.0394, -124.9023) -> (98.2131, -123.9175)
  line L406 (102.9635, -125.7705) -> (98.0394, -124.9023)
  line L407 (103.1371, -124.7857) -> (102.9635, -125.7705)
  line L408 (98.2131, -123.9175) -> (103.1371, -124.7857)
  line L409 (103.6667, -121.7821) -> (98.7427, -120.9138)
  line L410 (103.8404, -120.7973) -> (103.6667, -121.7821)
  line L411 (98.9163, -119.929) -> (103.8404, -120.7973)
  line L412 (98.7427, -120.9138) -> (98.9163, -119.929)
  line L413 (106.4451, -106.0251) -> (106.2715, -107.01)
  line L414 (101.5211, -105.1569) -> (106.4451, -106.0251)
  line L415 (106.2715, -107.01) -> (101.3474, -106.1417)
  line L416 (101.3474, -106.1417) -> (101.5211, -105.1569)
  line L417 (102.0507, -102.1532) -> (102.2243, -101.1684)
  line L418 (106.9747, -103.0215) -> (102.0507, -102.1532)
  line L419 (107.1484, -102.0367) -> (106.9747, -103.0215)
  line L420 (102.2243, -101.1684) -> (107.1484, -102.0367)
  line L421 (104.8291, -86.3963) -> (109.7531, -87.2646)
  line L422 (109.5795, -88.2494) -> (104.6554, -87.3811)
  line L423 (109.7531, -87.2646) -> (109.5795, -88.2494)
  line L424 (104.6554, -87.3811) -> (104.8291, -86.3963)
  line L425 (105.3587, -83.3927) -> (105.5323, -82.4078)
  line L426 (110.2827, -84.2609) -> (105.3587, -83.3927)
  line L427 (110.4564, -83.2761) -> (110.2827, -84.2609)
  line L428 (105.5323, -82.4078) -> (110.4564, -83.2761)
  line L429 (107.9634, -68.6205) -> (108.1371, -67.6357)
  line L430 (112.8875, -69.4888) -> (107.9634, -68.6205)
  line L431 (113.0611, -68.504) -> (112.8875, -69.4888)
  line L432 (108.1371, -67.6357) -> (113.0611, -68.504)
  line L433 (114.8031, -139.5356) -> (119.7271, -140.4038)
  line L434 (114.6294, -140.5204) -> (114.8031, -139.5356)
  line L435 (119.7271, -140.4038) -> (119.5534, -141.3886)
  line L436 (119.5534, -141.3886) -> (114.6294, -140.5204)
  line L437 (117.2341, -125.7483) -> (117.4078, -124.7635)
  line L438 (122.1582, -126.6165) -> (117.2341, -125.7483)
  line L439 (122.3318, -125.6317) -> (122.1582, -126.6165)
  line L440 (117.4078, -124.7635) -> (122.3318, -125.6317)
  line L441 (122.8614, -122.6281) -> (117.9374, -121.7598)
  line L442 (123.0351, -121.6432) -> (122.8614, -122.6281)
  line L443 (118.111, -120.775) -> (123.0351, -121.6432)
  line L444 (117.9374, -121.7598) -> (118.111, -120.775)
  line L445 (125.6398, -106.8711) -> (125.4662, -107.8559)
  line L446 (120.7158, -106.0029) -> (125.6398, -106.8711)
  line L447 (125.4662, -107.8559) -> (120.5421, -106.9877)
  line L448 (120.5421, -106.9877) -> (120.7158, -106.0029)
  line L449 (121.2454, -102.9992) -> (121.419, -102.0144)
  line L450 (126.1694, -103.8675) -> (121.2454, -102.9992)
  line L451 (126.3431, -102.8827) -> (126.1694, -103.8675)
  line L452 (121.419, -102.0144) -> (126.3431, -102.8827)
  line L453 (124.0238, -87.2423) -> (128.9478, -88.1105)
  line L454 (128.7742, -89.0953) -> (123.8501, -88.2271)
  line L455 (128.9478, -88.1105) -> (128.7742, -89.0953)
  line L456 (123.8501, -88.2271) -> (124.0238, -87.2423)
  line L457 (124.5534, -84.2386) -> (124.727, -83.2538)
  line L458 (129.4774, -85.1069) -> (124.5534, -84.2386)
  line L459 (129.6511, -84.1221) -> (129.4774, -85.1069)
  line L460 (124.727, -83.2538) -> (129.6511, -84.1221)
  line L461 (127.1581, -69.4665) -> (127.3318, -68.4817)
  line L462 (132.0822, -70.3348) -> (127.1581, -69.4665)
  line L463 (132.2558, -69.35) -> (132.0822, -70.3348)
  line L464 (127.3318, -68.4817) -> (132.2558, -69.35)
  line L465 (134.3451, -138.412) -> (139.2691, -139.2802)
  line L466 (134.1714, -139.3968) -> (134.3451, -138.412)
  line L467 (139.2691, -139.2802) -> (139.0954, -140.265)
  line L468 (139.0954, -140.265) -> (134.1714, -139.3968)
  line L469 (136.7761, -124.6246) -> (136.9498, -123.6398)
  line L470 (141.7002, -125.4929) -> (136.7761, -124.6246)
  line L471 (141.8738, -124.5081) -> (141.7002, -125.4929)
  line L472 (136.9498, -123.6398) -> (141.8738, -124.5081)
  line L473 (142.4034, -121.5044) -> (137.4794, -120.6362)
  line L474 (142.5771, -120.5196) -> (142.4034, -121.5044)
  line L475 (137.6531, -119.6514) -> (142.5771, -120.5196)
  line L476 (137.4794, -120.6362) -> (137.6531, -119.6514)
  line L477 (145.1818, -105.7475) -> (145.0082, -106.7323)
  line L478 (140.2578, -104.8793) -> (145.1818, -105.7475)
  line L479 (145.0082, -106.7323) -> (140.0841, -105.8641)
  line L480 (140.0841, -105.8641) -> (140.2578, -104.8793)
  line L481 (140.7874, -101.8756) -> (140.9611, -100.8908)
  line L482 (145.7114, -102.7438) -> (140.7874, -101.8756)
  line L483 (145.8851, -101.759) -> (145.7114, -102.7438)
  line L484 (140.9611, -100.8908) -> (145.8851, -101.759)
  line L485 (143.5658, -86.1187) -> (148.4898, -86.9869)
  line L486 (148.3162, -87.9717) -> (143.3921, -87.1035)
  line L487 (148.4898, -86.9869) -> (148.3162, -87.9717)
  line L488 (143.3921, -87.1035) -> (143.5658, -86.1187)
  line L489 (144.0954, -83.115) -> (144.2691, -82.1302)
  line L490 (149.0194, -83.9832) -> (144.0954, -83.115)
  line L491 (149.1931, -82.9984) -> (149.0194, -83.9832)
  line L492 (144.2691, -82.1302) -> (149.1931, -82.9984)
  line L493 (146.7001, -68.3429) -> (146.8738, -67.3581)
  line L494 (151.6242, -69.2111) -> (146.7001, -68.3429)
  line L495 (151.7978, -68.2263) -> (151.6242, -69.2111)
  line L496 (146.8738, -67.3581) -> (151.7978, -68.2263)
  line L497 (153.1056, -141.72) -> (158.0297, -142.5882)
  line L498 (152.932, -142.7048) -> (153.1056, -141.72)
  line L499 (158.0297, -142.5882) -> (157.856, -143.573)
  line L500 (157.856, -143.573) -> (152.932, -142.7048)
  line L501 (155.5367, -127.9326) -> (155.7104, -126.9478)
  line L502 (160.4608, -128.8009) -> (155.5367, -127.9326)
  line L503 (160.6344, -127.8161) -> (160.4608, -128.8009)
  line L504 (155.7104, -126.9478) -> (160.6344, -127.8161)
  line L505 (161.164, -124.8124) -> (156.24, -123.9442)
  line L506 (161.3377, -123.8276) -> (161.164, -124.8124)
  line L507 (156.4136, -122.9594) -> (161.3377, -123.8276)
  line L508 (156.24, -123.9442) -> (156.4136, -122.9594)
  line L509 (163.9424, -109.0555) -> (163.7688, -110.0403)
  line L510 (159.0184, -108.1872) -> (163.9424, -109.0555)
  line L511 (163.7688, -110.0403) -> (158.8447, -109.1721)
  line L512 (158.8447, -109.1721) -> (159.0184, -108.1872)
  line L513 (159.548, -105.1836) -> (159.7216, -104.1988)
  line L514 (164.472, -106.0518) -> (159.548, -105.1836)
  line L515 (164.6457, -105.067) -> (164.472, -106.0518)
  line L516 (159.7216, -104.1988) -> (164.6457, -105.067)
  line L517 (162.3264, -89.4267) -> (167.2504, -90.2949)
  line L518 (167.0768, -91.2797) -> (162.1527, -90.4115)
  line L519 (167.2504, -90.2949) -> (167.0768, -91.2797)
  line L520 (162.1527, -90.4115) -> (162.3264, -89.4267)
  line L521 (162.856, -86.423) -> (163.0296, -85.4382)
  line L522 (167.78, -87.2912) -> (162.856, -86.423)
  line L523 (167.9537, -86.3064) -> (167.78, -87.2912)
  line L524 (163.0296, -85.4382) -> (167.9537, -86.3064)
  line L525 (165.4607, -71.6509) -> (165.6344, -70.6661)
  line L526 (170.3848, -72.5191) -> (165.4607, -71.6509)
  line L527 (170.5584, -71.5343) -> (170.3848, -72.5191)
  line L528 (165.6344, -70.6661) -> (170.5584, -71.5343)
  line L529 (132.7854, -66.3463) -> (127.8614, -65.478)
  line L530 (127.8614, -65.478) -> (128.035, -64.4932)
  line L531 (132.9591, -65.3615) -> (132.7854, -66.3463)
  line L532 (128.035, -64.4932) -> (132.9591, -65.3615)
  line L533 (135.3902, -51.5742) -> (130.4661, -50.7059)
  line L534 (135.5638, -50.5894) -> (135.3902, -51.5742)
  line L535 (130.6398, -49.7211) -> (135.5638, -50.5894)
  line L536 (130.4661, -50.7059) -> (130.6398, -49.7211)
  line L537 (152.3274, -65.2227) -> (147.4034, -64.3544)
  line L538 (147.4034, -64.3544) -> (147.577, -63.3696)
  line L539 (152.5011, -64.2378) -> (152.3274, -65.2227)
  line L540 (147.577, -63.3696) -> (152.5011, -64.2378)
  line L541 (154.9322, -50.4505) -> (150.0081, -49.5823)
  line L542 (155.1058, -49.4657) -> (154.9322, -50.4505)
  line L543 (150.1818, -48.5975) -> (155.1058, -49.4657)
  line L544 (150.0081, -49.5823) -> (150.1818, -48.5975)
  line L545 (171.088, -68.5306) -> (166.164, -67.6624)
  line L546 (166.164, -67.6624) -> (166.3376, -66.6776)
  line L547 (171.2617, -67.5458) -> (171.088, -68.5306)
  line L548 (166.3376, -66.6776) -> (171.2617, -67.5458)
  line L549 (173.6927, -53.7585) -> (168.7687, -52.8903)
  line L550 (173.8664, -52.7737) -> (173.6927, -53.7585)
  line L551 (168.9424, -51.9055) -> (173.8664, -52.7737)
  line L552 (168.7687, -52.8903) -> (168.9424, -51.9055)
  line L553 (113.7028, -54.9566) -> (109.0043, -53.2465)
  line L554 (109.0043, -53.2465) -> (109.3464, -52.3068)
  line L555 (114.0448, -54.0169) -> (113.7028, -54.9566)
  line L556 (109.3464, -52.3068) -> (114.0448, -54.0169)
  line L557 (118.8331, -40.8612) -> (114.1346, -39.1511)
  line L558 (119.1751, -39.9216) -> (118.8331, -40.8612)
  line L559 (114.4767, -38.2115) -> (119.1751, -39.9216)
  line L560 (114.1346, -39.1511) -> (114.4767, -38.2115)
  line L561 (86.9566, -53.6058) -> (86.4566, -54.4718)
  line L562 (86.4566, -54.4718) -> (92.3022, -57.8468)
  line L563 (98.5784, -43.2261) -> (99.0784, -42.3601)
  line L564 (99.0784, -42.3601) -> (96.4804, -40.8601)
  line L565 (96.4804, -40.8601) -> (95.9804, -41.7261)
  line L566 (98.5784, -43.2261) -> (95.9804, -41.7261)
  line L567 (65.8452, -42.5718) -> (71.6908, -45.9468)
  line L568 (71.6908, -45.9468) -> (72.1908, -45.0808)
  line L569 (77.967, -31.3261) -> (78.467, -30.4601)
  line L570 (78.467, -30.4601) -> (75.869, -28.9601)
  line L571 (75.869, -28.9601) -> (75.369, -29.8261)
  line L572 (77.967, -31.3261) -> (75.369, -29.8261)
  line L573 (57.3241, -41.29) -> (58.0901, -41.9328)
  line L574 (58.0901, -41.9328) -> (53.7513, -47.1036)
  line L575 (68.2836, -28.2289) -> (69.0497, -28.8717)
  line L576 (69.0497, -28.8717) -> (73.3885, -23.7009)
  line L577 (44.7814, -33.2131) -> (44.0154, -32.5703)
  line L578 (44.0154, -32.5703) -> (42.087, -34.8684)
  line L579 (42.087, -34.8684) -> (42.853, -35.5112)
  line L580 (42.853, -35.5112) -> (44.7814, -33.2131)
  line L581 (60.0798, -14.9812) -> (59.3137, -14.3384)
  line L582 (59.3137, -14.3384) -> (57.3853, -16.6366)
  line L583 (57.3853, -16.6366) -> (58.1514, -17.2794)
  line L584 (58.1514, -17.2794) -> (60.0798, -14.9812)
  line L585 (63.0124, -62.2176) -> (63.9972, -62.3912)
  line L586 (63.9972, -62.3912) -> (65.1693, -55.7438)
  line L587 (59.8643, -85.8297) -> (61.0365, -79.1822)
  line L588 (61.0365, -79.1822) -> (60.0517, -79.0086)
  line L589 (44.63, -81.2395) -> (43.6452, -81.0659)
  line L590 (43.6452, -81.0659) -> (44.1661, -78.1114)
  line L591 (44.1661, -78.1114) -> (45.1509, -78.2851)
  line L592 (44.63, -81.2395) -> (45.1509, -78.2851)
  line L593 (49.2837, -54.8467) -> (48.2989, -54.673)
  line L594 (48.2989, -54.673) -> (47.778, -57.6274)
  line L595 (47.778, -57.6274) -> (48.7628, -57.8011)
  line L596 (48.7628, -57.8011) -> (49.2837, -54.8467)
  line L597 (15.275, -105.37) -> (8.525, -105.37)
  line L598 (8.525, -105.37) -> (8.525, -104.37)
  line L599 (15.275, -101.87) -> (13.55, -101.87)
  line L600 (15.275, -95.585) -> (15.275, -101.87)
  line L601 (8.525, -101.87) -> (8.525, -97.4)
  line L602 (-15.275, -105.37) -> (-8.525, -105.37)
  line L603 (-8.525, -105.37) -> (-8.525, -104.37)
  line L604 (-15.275, -101.87) -> (-15.275, -95.585)
  line L605 (-8.525, -97.4) -> (-8.525, -101.87)
  line L606 (-8.525, -101.87) -> (-10.25, -101.87)
  line L607 (13.4, -89.57) -> (10.4, -89.57)
  line L608 (10.4, -89.57) -> (10.4, -88.57)
  line L609 (10.4, -88.57) -> (13.4, -88.57)
  line L610 (13.4, -88.57) -> (13.4, -89.57)
  line L611 (-10.4, -89.57) -> (-13.4, -89.57)
  line L612 (-13.4, -89.57) -> (-13.4, -88.57)
  line L613 (-13.4, -88.57) -> (-10.4, -88.57)
  line L614 (-10.4, -88.57) -> (-10.4, -89.57)
  line L615 (8.525, -89.57) -> (15.275, -89.57)
  line L616 (-15.275, -89.57) -> (-8.525, -89.57)
  line L617 (86.9566, -53.6058) -> (72.1908, -45.0808)
  line L618 (65.8452, -42.5718) -> (69.8302, -35.6696)
  line L619 (69.8302, -35.6696) -> (96.2872, -50.9446)
  line L620 (92.3022, -57.8468) -> (96.2872, -50.9446)
  line L621 (85.5436, -34.003) -> (86.0436, -33.137)
  line L622 (90.3738, -35.637) -> (89.8738, -36.503)
  line L623 (89.8738, -36.503) -> (85.5436, -34.003)
  line L624 (86.0436, -33.137) -> (90.3738, -35.637)
  line L625 (48.7333, -26.2164) -> (47.9673, -25.5736)
  line L626 (51.1812, -21.7434) -> (51.9473, -22.3862)
  line L627 (51.9473, -22.3862) -> (48.7333, -26.2164)
  line L628 (47.9673, -25.5736) -> (51.1812, -21.7434)
  line L629 (53.7513, -47.1036) -> (47.6459, -41.9806)
  line L630 (47.6459, -41.9806) -> (67.2831, -18.5779)
  line L631 (67.2831, -18.5779) -> (73.3885, -23.7009)
  line L632 (68.2836, -28.2289) -> (57.3241, -41.29)
  line L633 (59.8643, -85.8297) -> (52.0154, -84.4457)
  line L634 (52.0154, -84.4457) -> (57.3204, -54.3598)
  line L635 (57.3204, -54.3598) -> (65.1693, -55.7438)
  line L636 (60.0517, -79.0086) -> (63.0124, -62.2176)
  line L637 (45.0751, -70.2498) -> (44.0903, -70.0762)
  line L638 (44.9585, -65.1522) -> (45.9433, -65.3258)
  line L639 (45.9433, -65.3258) -> (45.0751, -70.2498)
  line L640 (44.0903, -70.0762) -> (44.9585, -65.1522)
  line L641 (15.275, -105.37) -> (15.275, -97.4)
  line L642 (15.275, -97.4) -> (-15.275, -97.4)
  line L643 (-15.275, -97.4) -> (-15.275, -105.37)
  line L644 (-8.525, -104.37) -> (8.525, -104.37)
  line L645 (-7, -97.4) -> (-8.525, -97.4)
  line L646 (2.5, -88.1) -> (-2.5, -88.1)
  line L647 (-2.5, -87.1) -> (2.5, -87.1)
  line L648 (2.5, -87.1) -> (2.5, -88.1)
  line L649 (-2.5, -88.1) -> (-2.5, -87.1)
  line L650 (-7, -88.1) -> (7, -88.1)
  dimension "d504" = 2.7
  dimension "d508" = 2.7
  dimension "d510" = 3.675
  dimension "d511" = 3.825
  dimension "d514" = 2.7
  dimension "d515" = 2.7
  dimension "d516" = 2.7
  dimension "d517" = 1.35
  dimension "d518" = 1.35
  dimension "d519" = 1.35
  dimension "d520" = 2.7
  dimension "d563" = 4.5
  dimension "d564" = 5
  dimension "d565" = 1
  dimension "d566" = 14
  dimension "d567" = 19.05
  dimension "d568" = 4.5
  dimension "d569" = 14
  dimension "d570" = 19.05
  dimension "d571" = 19.05
  dimension "d572" = 14
  dimension "d614" = 4.5
  dimension "d638" = 4.5
  dimension "d639" = 4.5
  dimension "d640" = 4.5
  dimension "d641" = 4.5
  dimension "d642" = 4.5
  dimension "d643" = 4.5
  dimension "d644" = 4.5
  dimension "d674" = 3
  dimension "d676" = 1.875
  dimension "d678" = 1
  dimension "d679" = 1.875
  dimension "d680" = 1.875
  dimension "d681" = 1.875
  dimension "d682" = 1.875
  dimension "d683" = 1.875
  dimension "d684" = 1.875
  dimension "d685" = 1.875
  dimension "d687" = 3.5
  dimension "d688" = 1
  dimension "d689" = 4.5
  dimension "d690" = 4.5
  dimension "d691" = 1
  dimension "d692" = 3.5
  dimension "d693" = 3.5
  dimension "d694" = 1
  dimension "d695" = 4.5
  dimension "d696" = 3.5
  dimension "d697" = 1
  constraint perpendicular L43 L231
  constraint perpendicular L231 L232
  constraint perpendicular L228 L233
  constraint coincident L230.start L234.start
  constraint perpendicular L231 L234
  constraint coincident L229.end A0.end
  constraint perpendicular L233 L235
  constraint perpendicular L237 L240
  constraint parallel L237 L239
  constraint coincident A1.end L237.start
  constraint perpendicular L239 L241
  constraint parallel L231 L242
  constraint horizontal L243
  constraint perpendicular L243 L244
  constraint perpendicular L244 L245
  constraint parallel L238 L246
  constraint tangent L233 A3
  constraint tangent A3 A4
  constraint tangent L239 A4
  constraint coincident A0.start A1.start
  constraint collinear L148 L250
  constraint parallel L238 L252
  constraint perpendicular L238 L253
  constraint perpendicular L253 L254
  constraint coincident L252.start L255
  constraint coincident L254.end L255
  constraint horizontal L258
  constraint vertical L259
  constraint horizontal L260
  constraint vertical L261
  constraint equal L257 L258
  constraint equal L254 L259
  constraint collinear L254 L259
  constraint horizontal L262
  constraint vertical L263
  constraint horizontal L264
  constraint vertical L265
  constraint collinear L257 L262
  constraint equal L254 L265
  constraint equal L257 L262
  constraint horizontal L266
  constraint vertical L267
  constraint horizontal L268
  constraint vertical L269
  constraint collinear L263 L267
  constraint collinear L258 L266
  constraint equal L257 L266
  constraint equal L254 L269
  constraint horizontal L270
  constraint vertical L271
  constraint horizontal L272
  constraint vertical L273
  constraint equal L257 L272
  constraint equal L252 L271
  constraint collinear L270 L274
  constraint horizontal L276
  constraint vertical L277
  constraint horizontal L278
  constraint vertical L279
  constraint equal L270 L276
  constraint equal L271 L277
  constraint collinear L271 L277
  constraint horizontal L280
  constraint vertical L281
  constraint horizontal L282
  constraint vertical L283
  constraint collinear L272 L282
  constraint equal L271 L283
  constraint equal L272 L282
  constraint horizontal L284
  constraint vertical L285
  constraint horizontal L286
  constraint vertical L287
  constraint collinear L281 L285
  constraint collinear L276 L284
  constraint collinear L278 L286
  constraint collinear L283 L287
  constraint horizontal L288
  constraint vertical L289
  constraint horizontal L290
  constraint vertical L291
  constraint collinear L282 L290
  constraint collinear L280 L288
  constraint equal L282 L290
  constraint horizontal L292
  constraint vertical L293
  constraint horizontal L294
  constraint vertical L295
  constraint collinear L289 L293
  constraint collinear L291 L295
  constraint collinear L284 L292
  constraint collinear L286 L294
  constraint horizontal L296
  constraint vertical L297
  constraint horizontal L298
  constraint vertical L299
  constraint collinear L277 L297
  constraint collinear L279 L299
  constraint collinear L296 L300
  constraint equal L277 L297
  constraint horizontal L301
  constraint vertical L302
  constraint horizontal L303
  constraint vertical L304
  constraint collinear L285 L302
  constraint collinear L287 L304
  constraint collinear L298 L303
  constraint collinear L296 L301
  constraint horizontal L305
  constraint vertical L306
  constraint horizontal L307
  constraint vertical L308
  constraint collinear L293 L306
  constraint collinear L295 L308
  constraint collinear L303 L307
  constraint collinear L301 L305
  constraint horizontal L309
  constraint vertical L310
  constraint horizontal L311
  constraint vertical L312
  constraint collinear L297 L310
  constraint collinear L299 L312
  constraint equal L299 L312
  constraint horizontal L313
  constraint vertical L314
  constraint horizontal L315
  constraint vertical L316
  constraint collinear L304 L316
  constraint collinear L302 L314
  constraint collinear L309 L313
  constraint collinear L311 L315
  constraint horizontal L317
  constraint vertical L318
  constraint horizontal L319
  constraint vertical L320
  constraint collinear L308 L320
  constraint collinear L306 L318
  constraint collinear L313 L317
  constraint collinear L315 L319
  constraint collinear L25 L323